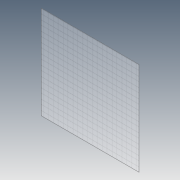
# Autodesk Inventor part: GE-12093
Saved by Autodesk Inventor 2012 (Build 160160000, 160)
## iProperties
Created: 2011-10-11
Part Number: GE-12093
Document SubType Name: Modeling
Designer: dfoster
Density: 1 g/cm^3
Description: Net, Corral Side
Material: Default
Title: Net, Corral Side
Author: dfoster
Autodesk Inventor part; units mm, degrees
ref_plane "YZ Plane" through (0, 0, 0) normal (1, 0, 0) x (0, 1, 0)
ref_plane "XZ Plane" through (0, 0, 0) normal (0, 1, 0) x (-1, 0, 0)
ref_plane "XY Plane" through (0, 0, 0) normal (0, 0, 1) x (1, 0, 0)
sketch "Sketch1" plane through (0, 0, 0) normal (0, 0, 1) x (1, 0, 0)
  line L0 (0, 0) -> (-1219.2, 0)
  line L1 (-1219.2, 0) -> (-1219.2, 1162.05)
  line L2 (-1219.2, 1162.05) -> (0, 1162.05)
  line L3 (0, 1162.05) -> (0, 0)
  dimension "d0" = 1219.2
  dimension "d1" = 1162.05
  constraints: 8 end point, 2 parallel, 1 horizontal, 1 perpendicular
  measures "d0" distance of L0.start L0.end
  measures "d1" distance of L2.end L0.start
extrude "Extrusion1" add sketch "Sketch1" along normal blind 3.175
body "Solid1"
